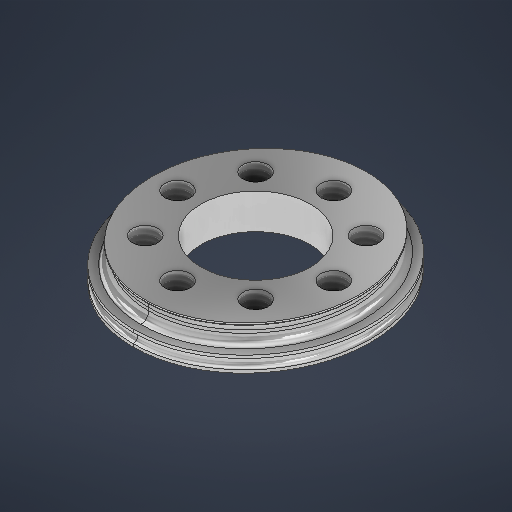
# Autodesk Inventor part: ELIPSE_DRIVE,REV-ENG
Saved by Autodesk Inventor 2026.2 (Build 302298010, 298A)
## iProperties
Created: 2026-03-06
Part Number: ELIPSE_DRIVE,REV-ENG
Material: Steel, 4140, Carb & Flame Harden 58-62 Rc
Document SubType Name: Modeling
Designer: 4aida
Density: 7.86 g/cm^3
Appearance: Chrome - Polished
Author: 4aida
Autodesk Inventor part; units mm, degrees
ref_plane "YZ Plane" through (0, 0, 0) normal (1, 0, 0) x (0, 1, 0)
ref_plane "XZ Plane" through (0, 0, 0) normal (0, 1, 0) x (-1, 0, 0)
ref_plane "XY Plane" through (0, 0, 0) normal (0, 0, 1) x (1, 0, 0)
sketch "Sketch1" plane through (0, 0, 0) normal (0, 1, 0) x (-1, 0, 0)
  ellipse E0 centre (0, 0) end of major axis (0, 16.2) minor radius 15.2
  dimension "d0" = 15.2
  dimension "d1" = 16.2
  constraints: 1 coincident, 2 other
sketch "Sketch2" plane through (0, 0, 0) normal (1, 0, 0) x (0, 1, 0)
  line L0 (-1.1125, 13.7) -> (-1.5, 13.7)
  line L1 (-2.5, 14.7) -> (-2.5, 15.7)
  line L2 (-4.5, 15.7) -> (-4.5, 8.7)
  line L3 (-4.5, 8.7) -> (0, 8.7)
  line L4 (0, 8.7) -> (0, 14.1857)
  arc A0 (-2.5, 14.7) -> (-1.5, 13.7) centre (-1.5, 14.7) ccw
  circle A1 centre (-1.25, 14.95) radius 1.25 construction
  line L5 (0, -16.2) -> (0, 16.2) construction
  line L6 (0, 16.2) -> (-3.6965, 16.2) construction
  arc A2 (-4.125, 15.7) -> (-2.875, 15.7) centre (-3.5, 15.7) ccw
  line L7 (-2.5, 15.7) -> (-2.875, 15.7)
  line L8 (-4.125, 15.7) -> (-4.5, 15.7)
  arc A3 (-0.2, 14.1857) -> (-0.283, 14.1415) centre (-0.2, 14.0857) ccw
  arc A4 (-1.1125, 13.7) -> (-0.283, 14.1415) centre (-1.1125, 14.7) ccw
  line L9 (-0.2, 14.1857) -> (0, 14.1857)
  point P0 (0, 0)
  dimension "d2" = 1
  dimension "d3" = 2.5
  dimension "d5" = 2
  dimension "d6" = 5
  dimension "d25" = 1.25
  dimension "d26" = 0.5
  dimension "d27" = 0.375
  dimension "d28" = 0.375
  dimension "d31" = 0.1
  dimension "d32" = 0.2
  dimension "d33" = 0.01
  constraints: 18 end point, 9 tangent, 8 perpendicular, 8 point on circle, 5 centre point, 2 horizontal, 1 equal radius, 1 horizontal alignment, 1 point on line
  measures "d2" radius of A0
  measures "d3" diameter of A1
  measures "d5" distance between parallel lines of L1 L2
  measures "d6" distance between parallel lines of L3 L0
  measures "d25" diameter of A2
  measures "d26" distance between parallel lines of L6 L8
  measures "d27" distance of L1.end L7.end
  measures "d28" distance of L8.start L2.start
  measures "d31" radius of A3
  measures "d32" distance from line of L4 A3.centre
sweep "Sweep1" add profiles "Sketch2" path "Sketch1"
sketch "Sketch5" plane through (0.0162, 0, -0.0003) normal (0, 1, 0) x (1, 0, 0)
  circle A0 centre (-0.0162, -0.0003) radius 7
  spline S0 degree 9 poles (-0.0162, -8.7003) (1.2416, -8.7003) (2.4994, -8.4371) (3.7267, -7.9105) (4.894, -7.1165) (5.9484, -6.0379) (6.7997, -4.7081) (7.3892, -3.1988) (7.9784, -0.0003) (7.3892, 3.1982) (6.7997, 4.7074) (5.9484, 6.0373) (4.894, 7.1158) (3.7267, 7.9099) (2.4994, 8.4365) (-0.0162, 8.9629) (-2.5318, 8.4365) (-3.7591, 7.9099) (-4.9264, 7.1158) (-5.9808, 6.0373) (-6.8321, 4.7074) (-7.4216, 3.1982) (-8.0108, -0.0003) (-7.4216, -3.1988) (-6.8321, -4.7081) (-5.9808, -6.0379) (-4.9264, -7.1165) (-3.7591, -7.9105) (-2.5318, -8.4371) (-1.274, -8.7003) (-0.0162, -8.7003) knots 0 0 0 0 0 0 0 0 0 0 0.25 0.25 0.25 0.25 0.25 0.25 0.25 0.5 0.5 0.5 0.5 0.5 0.5 0.5 0.75 0.75 0.75 0.75 0.75 0.75 0.75 1 1 1 1 1 1 1 1 1 1 projected
  dimension "d34" = 14
  constraints: 1 centre point, 1 coincident, 1 other
  measures "d34" diameter of A0
extrude "Extrusion2" add sketch "Sketch5" against normal up to surface (4.5 mm away)
sketch "Sketch6" plane through (0.0162, 0, -0.0003) normal (0, 1, 0) x (1, 0, 0)
  point P0 (-0.0162, -0.0003)
  point P1 (9.9838, -0.0003)
  dimension "d37" = 10
  constraints: 1 horizontal alignment
  measures "d37" distance of point (-0.016, 0) point (9.984, 0)
hole "Hole2" at (10, 0, 0) direction (0, -1, 0) diameter 3.242 depth 5
pattern_circular "Circular Pattern2" count 8 over 360 about axis through (0, 0, 0) along (0, -1, 0) of "Hole2"
equation "\"d28\" = d27"
body "Solid1"
